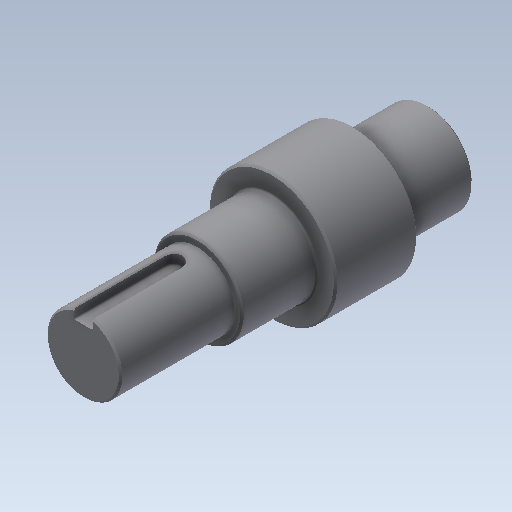
# Autodesk Inventor part: ShaftConfig_B_3.7_7.5.FDA658ECE0FAA460A03A372F46ED1B09
Saved by Autodesk Inventor 2021 (Build 250183000, 183)
## iProperties
Created: 2012-08-01
Material: Generic
Document SubType Name: Modeling
Designer: Parker Hannifin
Density: 1 g/cm^3
Part Number: ShaftConfig_B_3.7_7.5.FDA658ECE0FAA460A03A372F46ED1B09
Appearance: Default
Author: Parker Hannifin
Autodesk Inventor part; units mm, degrees
sketch "Sketch1" plane through (0, 0, 0) normal (0, 0, 1) x (1, 0, 0)
  line L0 (0, -22.225) -> (0, 22.225) construction
  line L1 (-22.225, 0) -> (22.225, 0) construction
  circle A0 centre (0, 0) radius 15.875
  dimension "d0" = 31.75
  constraints: 1 centre point, 1 coincident
  measures "d0" diameter of A0
extrude "Extrusion1" add sketch "Sketch1" along normal mid plane 48.4188
sketch "Sketch2" plane through (0, 0, 24.2094) normal (0, 0, 1) x (1, 0, 0)
  line L0 (0, -22.2499) -> (0, 22.3742) construction
  line L1 (-22.225, 0) -> (22.225, 0) construction
  line L2 (3.9497, 15.3758) -> (3.9497, 12.1666)
  line L3 (0, 11.4046) -> (3.1877, 11.4046)
  arc A0 (3.1877, 11.4046) -> (3.9497, 12.1666) centre (3.1877, 12.1666) ccw construction
  arc A1 (3.9497, 15.3758) -> (0, 15.875) centre (0, 0) ccw
  line L4 (-3.9497, 15.3758) -> (-3.9497, 12.1666)
  line L5 (0, 11.4046) -> (-3.1877, 11.4046)
  arc A2 (-3.9497, 12.1666) -> (-3.1877, 11.4046) centre (-3.1877, 12.1666) ccw construction
  arc A3 (0, 15.875) -> (-3.9497, 15.3758) centre (0, 0) ccw
  line L6 (-3.9497, 12.1666) -> (-3.9497, 11.4046)
  line L7 (-3.1877, 11.4046) -> (-3.9497, 11.4046)
  line L8 (3.9497, 12.1666) -> (3.9497, 11.4046)
  line L9 (3.1877, 11.4046) -> (3.9497, 11.4046)
  point P0 (0, -15.875)
  dimension "d4" = 3.9497
  dimension "d5" = 27.2796
  dimension "d6" = 1.524
  dimension "d7" = 15.875
  dimension "d8" = 15.875
  constraints: 16 end point, 8 point on circle, 6 perpendicular, 6 tangent, 4 centre point, 4 symmetric about line, 3 point on line, 1 coincident, 2 other
  measures "d4" distance between parallel lines of L0 L2
  measures "d5" distance from line of point (0, -15.875) L3
  measures "d6" diameter of A0
  measures "d7" distance of point (0, 0) point (0, -15.875)
  measures "d8" radius of A1
extrude "Extrusion2" cut sketch "Sketch2" against normal blind 38.1
sketch "Sketch5" plane through (-3.9497, 11.4046, 24.2094) normal (0, 1, 0) x (1, 0, 0)
  line L0 (7.8994, 38.1) -> (0, 38.1) projected
  line L1 (0, 0) -> (0, 38.1) construction
  line L2 (7.8994, 38.1) -> (7.8994, 0) construction
  arc A0 (7.8994, 38.1) -> (0, 38.1) centre (3.9497, 38.1) ccw
  constraints: 2 end point, 2 point on circle, 1 centre point, 1 midpoint
extrude "Extrusion4" cut sketch "Sketch5" along normal up to surface
fillet "Fillet1" radius 0.762 3 edges at (0, 11.4046, -17.8403) (3.9497, 11.4046, 5.1594) (-3.9497, 11.4046, 5.1594)
sketch "Sketch3" plane through (0, 0, -24.2094) normal (0, 0, -1) x (-1, 0, 0)
  circle A0 centre (0, 0) radius 15.875 projected
extrude "Extrusion3" add sketch "Sketch3" along normal blind 98.425
sketch "Sketch4" plane through (0, 0, 0) normal (1, 0, 0) x (0, 1, 0)
  line L0 (27.178, -56.7214) -> (27.178, -90.1224)
  line L1 (0, -147.2946) -> (0, 24.5491) construction
  line L2 (-24.4856, 0) -> (35.7886, 0) construction
  line L3 (15.875, -122.6344) -> (15.875, -17.8403) construction
  line L4 (15.875, -122.6344) -> (-15.875, -122.6344) construction
  line L5 (18.2753, -24.2094) -> (15.875, -24.2094)
  line L6 (26.416, -55.9594) -> (19.7993, -55.9594)
  line L7 (26.416, -90.8844) -> (19.7993, -90.8844)
  line L8 (15.875, -122.6344) -> (18.2753, -122.6344)
  line L9 (19.0373, -24.9714) -> (19.0373, -55.1974)
  line L10 (19.0373, -91.6464) -> (19.0373, -121.8724)
  line L11 (15.875, -24.2094) -> (15.875, -122.6344)
  arc A0 (19.0373, -55.1974) -> (19.7993, -55.9594) centre (19.7993, -55.1974) ccw
  arc A1 (19.7993, -90.8844) -> (19.0373, -91.6464) centre (19.7993, -91.6464) ccw
  line L12 (27.178, -56.7214) -> (26.416, -55.9594)
  line L13 (27.178, -90.1224) -> (26.416, -90.8844)
  line L14 (19.0373, -24.9714) -> (18.2753, -24.2094)
  line L15 (19.0373, -121.8724) -> (18.2753, -122.6344)
  point P0 (0, 0)
  point P1 (27.178, -55.9594)
  point P2 (27.178, -90.8844)
  point P3 (19.0373, -24.2094)
  point P4 (19.0373, -122.6344)
  dimension "d19" = 27.178
  dimension "d20" = 98.425
  dimension "d22" = 34.925
  dimension "d23" = 31.75
  dimension "d24" = 19.0373
  dimension "d25" = 0.762
  dimension "d26" = 0.762
  dimension "d27" = 0.762
  dimension "d28" = 0.762
  dimension "d29" = 0.762
  dimension "d30" = 0.762
  dimension "d31" = 0.762
  dimension "d32" = 0.762
  dimension "d33" = 0.762
  dimension "d34" = 0.762
  constraints: 24 end point, 11 point on line, 4 horizontal, 4 point on circle, 4 tangent, 4 vertical, 2 centre point, 1 collinear
  measures "d19" distance between parallel lines of L1 L0
  measures "d20" distance from line of L4 point (19.037, -24.209)
  measures "d22" distance of point (27.178, -55.959) point (27.178, -90.884)
  measures "d23" distance between parallel lines of L8 L7
  measures "d24" distance between parallel lines of L1 L9
  measures "d25" radius of A0
  measures "d26" radius of A1
  measures "d27" distance of L0.start point (27.178, -55.959)
  measures "d28" distance of L6.start point (27.178, -55.959)
  measures "d29" distance of L0.end point (27.178, -90.884)
  measures "d30" distance of L7.start point (27.178, -90.884)
  measures "d31" distance of L9.start point (19.037, -24.209)
  measures "d32" distance of L5.start point (19.037, -24.209)
  measures "d33" distance of L10.end point (19.037, -122.634)
  measures "d34" distance of L8.end point (19.037, -122.634)
revolve "Revolution1" add sketch "Sketch4" angle 360 about axis through (0, 0, -10) along (0, 0, 1)
chamfer "Chamfer1" distance 0.762 angle 45 2 edges at (-9.7292, -12.5443, 24.2094) (12.5443, 9.7292, 24.2094)
ref_plane "WP_H" through (0, 0, 0) normal (0, -1, 0) x (1, 0, 0)
ref_plane "WP_End" through (0, 0, -73.4219) normal (0, 0, -1) x (-1, 0, 0)
equation "\"d0\" = K_"
equation "\"d1\" = L_"
equation "\"d4\" = 0.5 * M_"
equation "\"d5\" = N_"
equation "\"d7\" = 0.5 * K_"
equation "\"d8\" = 0.5 * K_"
equation "\"d9\" = O_"
equation "\"d28\" = d27"
equation "\"d29\" = d27"
equation "\"d30\" = d29"
equation "\"d32\" = d31"
equation "\"d33\" = d31"
equation "\"d34\" = d33"
equation "\"K_\" = 31.75"
equation "\"L_\" = 48.41875"
equation "\"N_\" = 27.2796"
equation "\"O_\" = 38.1"
equation "\"M_\" = 7.8994"
equation "\"d3\" = K_"
body "Solid1"
